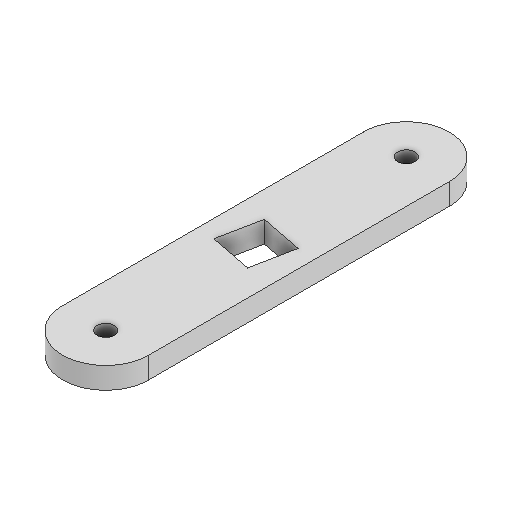
# Autodesk Inventor part: CameraAngle22.5
Saved by Autodesk Inventor 2025.2 (Build 292293000, 293)
## iProperties
Created: 2025-11-04
Part Number: CameraAngle22.5
Material: Generic
Document SubType Name: Modeling
Designer: rolan
Density: 1 g/cm^3
Appearance: Default
Author: rolan
Autodesk Inventor part; units mm, degrees
ref_plane "YZ Plane" through (0, 0, 0) normal (1, 0, 0) x (0, 1, 0)
ref_plane "XZ Plane" through (0, 0, 0) normal (0, 1, 0) x (-1, 0, 0)
ref_plane "XY Plane" through (0, 0, 0) normal (0, 0, 1) x (1, 0, 0)
sketch "Sketch1" plane through (0, 0, 0) normal (0, 1, 0) x (-1, 0, 0)
  line L0 (0, 35) -> (0, -35) construction
  line L1 (-10, 35) -> (-10, -35)
  line L2 (10, -35) -> (10, 35)
  arc A0 (10, 35) -> (-10, 35) centre (0, 35) ccw
  arc A1 (-10, -35) -> (10, -35) centre (0, -35) ccw
  circle A2 centre (0, -35) radius 2
  circle A3 centre (0, 35) radius 2
  line L3 (-5.8794, -3.9285) -> (-3.9285, 5.8794)
  line L4 (-3.9285, 5.8794) -> (5.8794, 3.9285)
  line L5 (5.8794, 3.9285) -> (3.9285, -5.8794)
  line L6 (3.9285, -5.8794) -> (-5.8794, -3.9285)
  line L7 (-5.8794, -3.9285) -> (5.8794, 3.9285) construction
  line L8 (-3.9285, 5.8794) -> (3.9285, -5.8794) construction
  line L9 (-5.8794, -3.9285) -> (4.1206, -3.9285) construction
  point P0 (0, 0)
  dimension "d0" = 35
  dimension "d1" = 20
  dimension "d2" = 4
  dimension "d3" = 4
  dimension "d4" = 10
  dimension "d5" = 78.75
  dimension "d6" = 10
  constraints: 22 end point, 4 centre point, 4 point on circle, 4 tangent, 3 midpoint, 3 parallel, 2 coincident, 1 equal length, 1 horizontal, 1 perpendicular, 1 vertical
  measures "d0" distance of point (0, 0) L0.end
  measures "d1" diameter of A1
  measures "d2" diameter of A2
  measures "d3" diameter of A3
  measures "d4" distance of L3.start L3.end
  measures "d5" angle of L9 L3
  measures "d6" distance of L3.end L4.end
extrude "Extrusion1" add sketch "Sketch1" along normal blind 5
body "Solid1"
